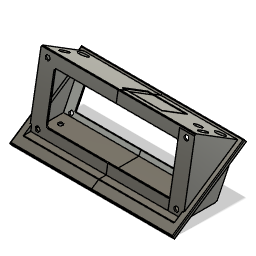
Trooper_Center_Gauges (Autodesk Fusion 360 design; units mm, degrees)
Autodesk Fusion 360 part; units mm, degrees
sketch "Base" plane through (0, 0, 0) normal (0, 1, 0) x (1, 0, 0)
  line L0 (101.6, -26.9875) -> (-101.6, -26.9875)
  line L1 (-101.6, -26.9875) -> (-101.6, 26.9875)
  line L2 (-101.6, 26.9875) -> (101.6, 26.9875)
  line L3 (101.6, 26.9875) -> (101.6, -26.9875)
  line L4 (101.6, -26.9875) -> (-101.6, 26.9875) construction
  line L5 (-101.6, -26.9875) -> (101.6, 26.9875) construction
  line L6 (-101.6, 11.7475) -> (101.6, 11.7475) construction
  circle A0 centre (-90.17, 11.7475) radius 3.175
  circle A1 centre (90.17, 11.7475) radius 3.175
  dimension "d1" = 203.2
  dimension "d2" = 53.975
  dimension "d3" = 15.24
  dimension "d4" = 6.35
  dimension "d5" = 6.35
  dimension "d6" = 11.43
  dimension "d7" = 11.43
  constraint horizontal L0
  constraint perpendicular L0 L1
  constraint parallel L0 L2
  constraint parallel L1 L3
  constraint coincident L4 origin
  constraint coincident L5 origin
  constraint coincident L1 L6.start
  constraint coincident L3 L6.end
  constraint perpendicular L3 L6
  constraint coincident L6 A0.centre
  constraint coincident L6 A1.centre
  measures "d1" distance of L1.end L2.end
  measures "d2" distance of L0.end L1.end
  measures "d3" distance of L2 L6
  measures "d4" diameter of A0
  measures "d5" diameter of A1
  measures "d6" distance of L6.start A0.centre
  measures "d7" distance of L6.end A1.centre
ref_plane "WorkPlane1" through (0, 0, -26.9875) normal (0, 0.438371, 0.898794) x (1, 0, 0)
sketch "Back" plane through (0, 0, -26.9875) normal (0, 0.438371, 0.898794) x (1, 0, 0)
  line L0 (-101.6, 0) -> (101.6, 0)
  line L1 (101.6, 0) -> (101.6, 60.325)
  line L2 (101.6, 60.325) -> (-101.6, 60.325)
  line L3 (-101.6, 60.325) -> (-101.6, 0)
  line L4 (-101.6, 0) -> (101.6, 0)
  line L5 (-88.9, 53.975) -> (88.9, 53.975)
  line L6 (88.9, 53.975) -> (88.9, 6.35)
  line L7 (88.9, 6.35) -> (-88.9, 6.35)
  line L8 (-88.9, 6.35) -> (-88.9, 53.975)
  line L9 (-101.6, 0) -> (101.6, 0)
  line L10 (101.6, 0) -> (101.6, -2.286)
  line L11 (101.6, -2.286) -> (-101.6, -2.286)
  line L12 (-101.6, -2.286) -> (-101.6, 0)
  point P0 (-101.6, 0)
  dimension "d9" = 60.325
  dimension "d10" = 12.7
  dimension "d11" = 12.7
  dimension "d12" = 6.35
  dimension "d13" = 6.35
  dimension "d28" = 2.286
  constraint horizontal L0
  constraint vertical L1
  constraint horizontal L2
  constraint vertical L3
  constraint coincident L0.end L1.start
  constraint horizontal L5
  constraint vertical L6
  constraint horizontal L7
  constraint vertical L8
  constraint coincident P0 L0.start
  constraint horizontal L9
  constraint vertical L10
  constraint horizontal L11
  constraint vertical L12
  measures "d9" distance of L2 L4
  measures "d10" distance of L3 L8
  measures "d11" distance of L1 L6
  measures "d12" distance of L2 L5
  measures "d13" distance of L0 L7
  measures "d28" distance of L9 L11
ref_plane "WorkPlane2" through (101.6, 54.2198, -53.4322) normal (0, -0.829153, -0.559022) x (1, 0, 0)
sketch "Trim" plane through (101.6, 54.2198, -53.4322) normal (0, -0.829153, -0.559022) x (1, 0, 0)
  line L0 (-203.2, 0) -> (0, 0)
  line L1 (0, 0) -> (0, 96.9903)
  line L2 (0, 96.9903) -> (-203.2, 96.9903)
  line L3 (-203.2, 96.9903) -> (-203.2, 0)
  line L4 (-211.455, -6.985) -> (8.255, -6.985)
  line L5 (8.255, -6.985) -> (8.255, 109.6903)
  line L6 (8.255, 109.6903) -> (-211.455, 109.6903)
  line L7 (-211.455, 109.6903) -> (-211.455, -6.985)
  point P0 (-203.2, 0)
  point P1 (0, 96.9903)
  point P2 (-203.2, 96.9903)
  point P3 (-203.2, 0)
  dimension "d14" = 8.255
  dimension "d15" = 8.255
  dimension "d16" = 6.985
  dimension "d17" = 12.7
  constraint horizontal L0
  constraint vertical L1
  constraint horizontal L2
  constraint vertical L3
  constraint horizontal L4
  constraint vertical L5
  constraint horizontal L6
  constraint vertical L7
  constraint coincident P2 L2.end
  constraint coincident P1 L1.end
  constraint coincident P3 P0
  measures "d14" distance of L3 L7
  measures "d15" distance of L1 L5
  measures "d16" distance of L0 L4
  measures "d17" distance of L2 L6
ref_plane "WorkPlane3" through (101.6, 0, -26.9875) normal (1, 0, 0) x (0, 1, 0)
sketch "Right" plane through (101.6, 0, -26.9875) normal (1, 0, 0) x (0, 0, -1)
  line L0 (-53.975, 0) -> (26.4447, 54.2198)
  line L1 (0, -2.032) -> (-53.975, -2.032)
  line L2 (-53.975, -2.032) -> (-53.975, 0)
  line L3 (1.8263, -0.8908) -> (28.2711, 53.329)
  line L4 (28.2711, 53.329) -> (26.4447, 54.2198)
  line L5 (0, -2.032) -> (1.8263, -0.8908)
  point P0 (26.4447, 54.2198)
  point P1 (-53.975, 0)
  dimension "d39" = 2.032
  dimension "d40" = 2.032
  constraint coincident P1 L0.start
  constraint coincident P0 L0.end
  measures "d39" distance of P1 L1.end
  measures "d40" distance of P0 L3.end
ref_plane "WorkPlane4" through (-101.6, 0, 26.9875) normal (-1, 0, 0) x (0, -1, 0)
sketch "Left" plane through (-101.6, 0, 26.9875) normal (-1, 0, 0) x (0, -1, 0)
  line L0 (0, 0) -> (-54.2198, -80.4197)
  line L1 (0.8908, -55.8013) -> (-53.329, -82.2461)
  line L2 (-53.329, -82.2461) -> (-54.2198, -80.4197)
  line L3 (2.032, -53.975) -> (2.032, 0)
  line L4 (2.032, 0) -> (0, 0)
  line L5 (0.8908, -55.8013) -> (2.032, -53.975)
  point P0 (0, -53.975)
  point P1 (-54.2198, -80.4197)
  dimension "d37" = 2.032
  dimension "d38" = 2.032
  constraint coincident L0.start L4.end
  constraint coincident P1 L0.end
  measures "d37" distance of P1 L1.end
  measures "d38" distance of L0.start L3.end
extrude "Extrude1" add sketch "Trim" along normal blind 4.572 makes body 1
extrude "Extrude2" add sketch "Back" against normal blind 2.032 contours L0 L1 L2 L3 L4 L9 bodies 1
extrude "Extrude3" add sketch "Base" against normal blind 2.032 bodies 1
extrude "Extrude4" add sketch "Right" along normal blind 2.032 bodies 1
extrude "Extrude5" add sketch "Left" along normal blind 2.032 bodies 1
extrude "Extrude6" add sketch "Back" against normal blind 2.032 contours L0 L4 L9 L10 L11 L12 bodies 1
fillet "Fillet1" radius 2.54 1 edges at (0, -2.9454, -27.8117) on bodies 1
fillet "Fillet2" radius 1.27 1 edges at (0, 0, 26.9875) on bodies 1
fillet "Fillet3" radius 1.016 4 edges at (0, -7.0996, 37.5177) (-109.855, 25.5125, -10.8531) (0, 58.1245, -59.2239) (109.855, 25.5125, -10.8531) on bodies 1
sketch "Left Tabs" plane through (-101.6, 0, 0) normal (1, 0, 0) x (0, 0, -1)
  line L0 (26.9875, 0) -> (49.4252, 46.0041)
  line L1 (49.4252, 46.0041) -> (-18.8089, 0)
  line L2 (-18.8089, 0) -> (26.9875, 0)
  line L3 (-26.67, 0) -> (-17.1035, 0) construction
  line L4 (-17.1035, 0) -> (1.1317, 103.4174) construction
  line L5 (-17.1035, 0) -> (-14.8982, 12.5071)
  line L6 (-14.8982, 12.5071) -> (-12.8971, 12.1542)
  line L7 (-12.8971, 12.1542) -> (-15.1024, -0.3529)
  line L8 (-15.1024, -0.3529) -> (-17.1035, 0)
  line L9 (-17.1035, 0) -> (-16.0009, 6.2535) construction
  line L10 (-16.0009, 6.2535) -> (-2.4932, 82.8593) construction
  line L11 (-2.4932, 82.8593) -> (-1.3905, 89.1128) construction
  line L12 (-1.3905, 89.1128) -> (-3.5959, 76.6057)
  line L13 (-3.5959, 76.6057) -> (-1.5947, 76.2529)
  line L14 (-1.5947, 76.2529) -> (0.6106, 88.7599)
  line L15 (0.6106, 88.7599) -> (-1.3905, 89.1128)
  line L16 (-26.9875, 0) -> (53.4322, 54.2198)
  line L17 (53.4322, 54.2198) -> (0.6106, 88.7599)
  line L18 (-1.5947, 76.2529) -> (-13.4282, 9.1418)
  line L19 (0.6106, 88.7599) -> (53.4322, 54.2198)
  line L20 (53.4322, 54.2198) -> (-27.3093, -0.217)
  line L21 (-27.3093, -0.217) -> (53.4322, 54.2198)
  line L22 (-36.6753, -6.5316) -> (58.3815, 57.5566)
  line L23 (58.3815, 57.5566) -> (-36.6753, -6.5316)
  line L24 (53.4322, 54.2198) -> (56.4461, 56.2518)
  line L25 (0.6106, 88.7599) -> (0.9634, 90.7611)
  line L26 (0.9634, 90.7611) -> (56.4461, 56.2518)
  line L27 (-1.3905, 89.1128) -> (-1.0377, 91.1139)
  line L28 (-1.0377, 91.1139) -> (0.9634, 90.7611)
  line L29 (-3.5959, 76.6057) -> (-14.8982, 12.5071)
  point P0 (55.2586, 53.329)
  point P1 (53.4322, 54.2198)
  point P2 (53.4322, 54.2197)
  point P3 (-36.6753, -6.5316)
  dimension "d41" = 12.7
  dimension "d42" = 2.032
  dimension "d43" = 77.7875
  dimension "d44" = 6.35
  dimension "d45" = 12.7
  dimension "d46" = 2.032
  dimension "d69" = 2.032
  dimension "d70" = 2.032
  dimension "d71" = 2.032
  dimension "d99" = 80
  dimension "d100" = 1.7054
  constraint coincident L2 L3.end
  constraint perpendicular L5 L6
  constraint parallel L5 L7
  constraint parallel L6 L8
  constraint parallel L4 L5
  constraint midpoint L5 L9.end
  constraint parallel L4 L10
  constraint parallel L4 L11
  constraint perpendicular L12 L13
  constraint parallel L12 L14
  constraint parallel L13 L15
  constraint parallel L4 L12
  constraint coincident P1 L16.end
  constraint coincident L16 L18.end
  constraint perpendicular L13 L18
  constraint coincident L22 L24.end
  constraint perpendicular L15 L25
  constraint perpendicular L15 L27
  measures "d41" distance of L3.end L5.end
  measures "d42" distance of L4 L7
  measures "d43" distance of L9.end L10.end
  measures "d44" distance of L10.end L11.end
  measures "d45" distance of L11.end L12.end
  measures "d46" distance of L10 L14
  measures "d69" vertical distance of P1 L24.end
  measures "d70" distance of L14.end L25.end
  measures "d71" distance of L11.end L27.end
  measures "d99" angle of L2 L4
  measures "d100" distance of L1.end L3.end
extrude "Extrude7" add sketch "Left Tabs" against normal blind 2.032 contours L5 L6 L7 L16 L18 L20 L21 L22 L23 | L7 L14 L16 L17 L18 L19 L20 L21 L22 L23 bodies 1
extrude "Extrude8" add sketch "Left Tabs" along normal blind 18.288 and the other way blind 2.032 contours L1 L2 L5 L7 | L1 L5 L7 L16 L20 L21 L22 L23 | L5 L6 L7 L16 L18 L20 L21 L22 L23 | L12 L13 L14 L15 bodies 1
sketch "Right Tabs" plane through (101.6, 0, 0) normal (-1, 0, 0) x (0, 0, 1)
  line L0 (-26.9875, 0) -> (26.5994, 0)
  arc A0 (27.3093, -0.217) -> (26.5994, 0) centre (26.5994, -1.27) ccw
  line L1 (27.3093, -0.217) -> (-53.4322, 54.2198)
  line L2 (-53.4322, 54.2198) -> (-26.9875, 0)
  line L3 (-53.4322, 54.2198) -> (-0.6106, 88.7599)
  line L4 (1.5947, 76.2529) -> (-0.6106, 88.7599)
  line L5 (1.5947, 76.2529) -> (13.4282, 9.1418)
  line L6 (-0.6106, 88.7599) -> (1.3905, 89.1128)
  line L7 (2.4932, 82.8593) -> (1.3905, 89.1128)
  line L8 (1.3905, 89.1128) -> (3.5959, 76.6057)
  line L9 (17.1035, 0) -> (-1.1317, 103.4174)
  line L10 (3.5959, 76.6057) -> (1.5947, 76.2529)
  line L11 (14.8982, 12.5071) -> (12.8971, 12.1542)
  line L12 (12.8971, 12.1542) -> (15.1024, -0.3529)
  line L13 (15.1024, -0.3529) -> (17.1035, 0)
  line L14 (17.1035, 0) -> (16.0009, 6.2535)
  line L15 (-1.1317, 103.4174) -> (17.1035, 0) construction
  line L16 (17.1035, 0) -> (16.0009, 6.2535) construction
  line L17 (16.0009, 6.2535) -> (2.4932, 82.8593) construction
  line L18 (2.4932, 82.8593) -> (1.3905, 89.1128) construction
  line L19 (2.4932, 82.8593) -> (3.5959, 76.6057) construction
  line L20 (-53.4322, 54.2198) -> (-0.6106, 88.7599)
  line L21 (1.3905, 89.1128) -> (3.5959, 76.6057)
  line L22 (3.5959, 76.6057) -> (1.5947, 76.2529)
  line L23 (1.5947, 76.2529) -> (-0.6106, 88.7599)
  line L24 (-0.6106, 88.7599) -> (1.3905, 89.1128)
  line L25 (14.8982, 12.5071) -> (17.1035, 0)
  line L26 (17.1035, 0) -> (15.1024, -0.3529)
  line L27 (15.1024, -0.3529) -> (12.8971, 12.1542)
  line L28 (12.8971, 12.1542) -> (14.8982, 12.5071)
  line L29 (1.5947, 76.2529) -> (13.4282, 9.1418)
  line L30 (3.5959, 76.6057) -> (14.8982, 12.5071)
  dimension "d101" = 2.032
  dimension "d102" = 2.032
  constraint coincident L9.end L15.start
  constraint coincident L9.start L13.end
  constraint coincident L14.end L16.end
  constraint coincident L7.start L17.end
  constraint coincident L6.end L7.end
  constraint coincident L8.end L10.start
  constraint coincident L1.end L2.start
  constraint coincident L3.end L4.end
  constraint perpendicular L21 L22
  constraint parallel L21 L23
  constraint parallel L22 L24
  constraint perpendicular L25 L26
  constraint parallel L25 L27
  constraint parallel L26 L28
  constraint perpendicular L13 L25
  constraint coincident L11.start L25.start
  constraint coincident L4.start L5.start
  constraint coincident L5.end L29.end
  measures "d101" distance of L18 L23
  measures "d102" distance of L15 L27
extrude "Extrude9" add sketch "Right Tabs" against normal blind 2.032 contours L1 L5 L9 L11 L12 L25 L27 L28 L29 | L1 L3 L4 L5 L12 L20 L23 L27 L29 | L5 L9 L10 L11 L22 L28 L29 L30 bodies 1
extrude "Extrude10" add sketch "Right Tabs" along normal blind 18.288 and the other way blind 2.032 contours L0 L1 L9 L12 L14 L25 L27 | L1 L5 L9 L11 L12 L25 L27 L28 L29 | L4 L6 L7 L8 L9 L10 L21 L22 L23 L24 bodies 1
extrude "Extrude12" add sketch "Left Tabs" along normal up to surface (205.232 mm away) contours L17 L19 L22 L23 L24 L25 L26 | L15 L25 L27 L28 bodies 1
ref_plane "WorkPlane5" through (-93.472, 82.5064, 0.4921) normal (0, 0.173648, 0.984808) x (0, -0.984808, 0.173648)
sketch "Tab Mounting Holes" plane through (0, 2.9249, 16.5878) normal (0, 0.173648, 0.984808) x (1, 0, 0)
  line L0 (-103.632, 74.8175) -> (-83.312, 74.8175)
  line L1 (-83.312, 74.8175) -> (-83.312, 87.5175)
  line L2 (-101.6, 87.5175) -> (-103.632, 87.5175)
  line L3 (-103.632, 87.5175) -> (-103.632, 74.8175)
  line L4 (83.312, 87.5175) -> (83.312, 74.8175)
  line L5 (83.312, 74.8175) -> (101.6, 74.8175)
  line L6 (103.632, 4.7096) -> (103.632, 87.5175)
  line L7 (-101.6, 4.7097) -> (-101.6, -1.6449)
  line L8 (-101.6, -1.6449) -> (-101.6, -2.97)
  line L9 (-101.6, -2.97) -> (-83.312, -2.97)
  line L10 (-83.312, -2.97) -> (-83.312, 9.73)
  line L11 (-83.312, 9.73) -> (-103.632, 9.73)
  line L12 (101.6, 74.8175) -> (101.6, 9.73)
  line L13 (83.312, 87.5175) -> (83.312, 74.8175)
  line L14 (83.312, -2.97) -> (101.6, -2.97)
  line L15 (-103.632, 9.73) -> (-83.312, -2.97) construction
  circle A0 centre (-93.472, 81.1675) radius 3.175
  circle A1 centre (-93.472, 3.38) radius 3.175
  line L16 (-83.312, 87.5175) -> (83.312, 87.5175)
  line L17 (83.312, 87.5175) -> (103.632, 87.5175)
  line L18 (103.632, 87.5175) -> (103.632, 89.5495)
  line L19 (103.632, 89.5495) -> (-101.6, 89.5495)
  line L20 (-101.6, 89.5495) -> (-101.6, 87.5175)
  line L21 (103.632, 87.5175) -> (83.312, 87.5175)
  line L22 (101.6, 74.8175) -> (101.6, 9.73)
  line L23 (101.6, 4.7096) -> (103.632, 4.7096)
  line L24 (101.6, 74.8175) -> (103.632, 74.8175) construction
  line L25 (-103.632, 9.73) -> (-103.632, 4.7097)
  line L26 (-103.632, 4.7096) -> (-101.6, 4.7096)
  line L27 (101.6, 9.73) -> (83.312, 9.73)
  line L28 (83.312, 9.73) -> (83.312, -2.97)
  line L29 (83.312, -2.97) -> (101.6, -2.97)
  line L30 (101.6, -2.97) -> (101.6, 4.7096)
  line L31 (103.632, 4.7096) -> (103.632, 87.5175)
  line L32 (103.632, 87.5175) -> (83.312, 87.5175)
  line L33 (83.312, 74.8175) -> (101.6, 74.8175)
  line L34 (101.6, 9.73) -> (83.312, 9.73)
  line L35 (83.312, 9.73) -> (83.312, -2.97)
  line L36 (101.6, -2.97) -> (101.6, 4.7096)
  line L37 (101.6, 4.7096) -> (103.632, 4.7096)
  line L38 (-83.312, 74.8175) -> (-103.632, 87.5175) construction
  line L39 (-83.312, 87.5175) -> (-103.632, 74.8175) construction
  line L40 (103.632, 87.5175) -> (83.312, 74.8175) construction
  line L41 (83.312, 87.5175) -> (103.632, 74.8175) construction
  line L42 (-101.6, -2.97) -> (-103.632, -2.97) construction
  line L43 (-103.632, -2.97) -> (-103.632, 4.7096) construction
  line L44 (101.6, -2.97) -> (103.632, -2.97) construction
  line L45 (103.632, 4.7096) -> (103.632, -2.97) construction
  line L46 (83.312, 9.73) -> (103.632, -2.97) construction
  line L47 (101.6, 9.73) -> (103.632, 9.73) construction
  line L48 (83.312, -2.97) -> (103.632, 9.73) construction
  line L49 (-83.312, 9.73) -> (-103.632, -2.97) construction
  circle A2 centre (93.472, 81.1675) radius 3.175
  circle A3 centre (93.472, 3.38) radius 3.175
  point P0 (-93.472, 3.38)
  point P1 (-93.472, 81.1675)
  point P2 (93.472, 81.1675)
  point P3 (93.472, 3.38)
  dimension "d60" = 77.7875
  dimension "d62" = 6.35
  dimension "d63" = 6.35
  dimension "d104" = 2.032
  dimension "d105" = 2.032
  dimension "d106" = 2.032
  dimension "d107" = 6.35
  dimension "d108" = 6.35
  constraint coincident L11.end L15.start
  constraint coincident L9.end L10.start
  constraint midpoint L15 P0
  constraint coincident P1 A0.centre
  constraint coincident P0 A1.centre
  constraint coincident L5.end L12.start
  constraint coincident L6 L24.end
  constraint perpendicular L6 L24
  constraint coincident L0.end L1.start
  constraint coincident L2.end L3.start
  constraint coincident L1.end L16.start
  constraint coincident L0.start L3.end
  constraint coincident L6.end L17.end
  constraint coincident L4.end L5.start
  constraint coincident L4.start L13.start
  constraint midpoint L41 P2
  constraint coincident L8.end L9.start
  constraint perpendicular L8 L42
  constraint coincident L26.start L43.end
  constraint coincident L14.end L29.end
  constraint perpendicular L30 L44
  constraint coincident L6.start L23.end
  constraint coincident L27.end L28.start
  constraint coincident L12.end L22.end
  constraint perpendicular L6 L47
  constraint coincident L14.start L28.end
  constraint coincident L10.end L11.start
  constraint midpoint L46 P3
  constraint coincident P2 A2.centre
  constraint coincident P3 A3.centre
  measures "d60" vertical distance of P0 P1
  measures "d62" diameter of A0
  measures "d63" diameter of A1
  measures "d104" distance of L8.end L42.end
  measures "d105" distance of L14.end L44.end
  measures "d106" distance of L12.end L47.end
  measures "d107" diameter of A2
  measures "d108" diameter of A3
extrude "Extrude11" cut sketch "Tab Mounting Holes" against normal blind 2.032 contours A0 | A1 | A2 | A3 bodies 1
extrude "Extrude20" cut sketch "Tab Mounting Holes" against normal through all contours A0 | A2 bodies 1
extrude "Extrude13" add sketch "Left Tabs" against normal up to surface (2.032 mm away) contours L17 L19 L22 L23 L24 L25 L26 | L15 L25 L27 L28 bodies 1
sketch "Screwdriver Holes - Back" plane through (0, -11.524, -23.6277) normal (0, -0.438371, -0.898794) x (-1, 0, 0)
  line L0 (-103.632, 12.0332) -> (101.6, 12.0332)
  line L1 (101.6, 12.0332) -> (101.6, 66.5327)
  line L2 (101.6, 66.5327) -> (101.6, 70.9818)
  line L3 (101.6, 70.9818) -> (-101.6, 70.9818)
  line L4 (-101.6, 70.9818) -> (-101.6, 66.5327)
  line L5 (-101.6, 66.5327) -> (-103.632, 66.5327)
  line L6 (-103.632, 66.5327) -> (-103.632, 12.0332)
  line L7 (88.9, 18.1805) -> (-88.9, 18.1805)
  line L8 (-88.9, 18.1805) -> (-88.9, 65.8055)
  line L9 (-88.9, 65.8055) -> (88.9, 65.8055)
  line L10 (88.9, 65.8055) -> (88.9, 18.1805)
  line L11 (-92.964, 15.24) -> (92.7862, 15.24) construction
  circle A0 centre (-92.964, 15.24) radius 2.794
  circle A1 centre (92.7862, 15.24) radius 2.794
  dimension "d111" = 185.7502
  dimension "d113" = 4.064
  dimension "d114" = 5.588
  dimension "d115" = 5.588
  constraint perpendicular L8 L11
  constraint coincident L11.start A0.centre
  constraint coincident L11.end A1.centre
  measures "d111" distance of L11.start L11.end
  measures "d113" horizontal distance of L7.end L11.start
  measures "d114" diameter of A0
  measures "d115" diameter of A1
extrude "Extrude21" cut sketch "Screwdriver Holes - Back" against normal blind 2.032 contours A0 | A1 bodies 1
ref_plane "WorkPlane6" through (0, 0, -11.7475) normal (0, -0.45399, -0.891007) x (1, 0, 0)
ref_plane "WorkPlane7" through (0, 73.5064, -28.7048) normal (0, 0.849148, -0.528156) x (0, 0.528156, 0.849148)
sketch "Screwdriver Holes - Top" plane through (0, 73.5064, -28.7048) normal (0, 0.849148, -0.528156) x (0, 0.528156, 0.849148)
  line L0 (32.6696, 103.632) -> (-32.6696, 103.632)
  line L1 (-32.6696, -103.632) -> (32.6696, -103.632)
  line L2 (-18.3286, 180.8064) -> (-18.3286, -180.8064)
  line L3 (-18.3286, 103.632) -> (-18.3286, 92.202) construction
  line L4 (-18.3286, -103.632) -> (-18.3286, -92.202) construction
  circle A0 centre (-18.3286, -92.202) radius 6.35
  circle A1 centre (-18.3286, 92.202) radius 6.35
  point P0 (-24.4236, 90.17)
  point P1 (-24.4236, -90.17)
  dimension "d78" = 11.43
  dimension "d79" = 11.43
  dimension "d80" = 12.7
  dimension "d81" = 12.7
  constraint coincident L2 L3.start
  constraint coincident L0 L3.start
  constraint coincident L2 L3.end
  constraint coincident L1 L4.start
  constraint coincident L2 L4.start
  constraint coincident L2 L4.end
  constraint coincident L4.end A0.centre
  constraint coincident L3.end A1.centre
  measures "d78" distance of L3.start L3.end
  measures "d79" distance of L4.start L4.end
  measures "d80" diameter of A0
  measures "d81" diameter of A1
extrude "Extrude14" cut sketch "Screwdriver Holes - Top" along normal up to surface end surface through (-101.6, 54.2198, -53.4322) normal (0, -0.836948, 0.547282) offset 0 bodies 1
sketch "Tab Connector Left" plane through (0, 73.6809, -12.9919) normal (0, -0.984808, 0.173648) x (1, 0, 0)
  line L0 (-101.6, 14.8117) -> (-83.312, 14.8117)
  line L1 (-83.312, 14.8117) -> (-83.312, 16.8437)
  line L2 (-83.312, 16.8437) -> (-103.632, 16.8437)
  line L3 (-103.632, 14.8117) -> (-101.6, 14.8117)
  line L4 (-103.632, 16.8437) -> (-103.632, 14.8117)
sketch "Tab Connector Bottom" plane through (-83.312, 0, 0) normal (1, 0, 0) x (0, 0, -1)
  line L0 (-17.1035, 0) -> (-15.0402, 0)
  line L1 (-15.0402, 0) -> (-12.8971, 12.1542)
  line L2 (-12.8971, 12.1542) -> (-14.8982, 12.5071)
  line L3 (-14.8982, 12.5071) -> (-17.1035, 0)
sketch "Tab Connector Top" plane through (-83.312, 0, 0) normal (1, 0, 0) x (0, 0, -1)
  line L0 (0.6106, 88.7599) -> (-1.3905, 89.1128)
  line L1 (-1.3905, 89.1128) -> (-3.5959, 76.6057)
  line L2 (-3.5959, 76.6057) -> (-1.5947, 76.2529)
  line L3 (-1.5947, 76.2529) -> (0.6106, 88.7599)
sketch "Tab Connector Right" plane through (0, 73.6809, -12.9919) normal (0, -0.984808, 0.173648) x (1, 0, 0)
  line L0 (101.6, 14.8117) -> (101.6, 16.8437)
  line L1 (101.6, 16.8437) -> (83.312, 16.8437)
  line L2 (83.312, 14.8117) -> (101.6, 14.8117)
  line L3 (83.312, 16.8437) -> (83.312, 14.8117)
extrude "Extrude16" add sketch "Tab Connector Bottom" along normal up to surface (166.624 mm away) bodies 1
extrude "Extrude19" add sketch "Tab Connector Left" along normal up to surface (65.0875 mm away) bodies 1
extrude "Extrude17" add sketch "Tab Connector Top" along normal up to surface (166.624 mm away) bodies 1
extrude "Extrude18" add sketch "Tab Connector Right" along normal up to surface (65.0875 mm away) bodies 1
fillet "Fillet5" radius 2.54 4 edges at (-83.312, 76.4293, 2.5953) (83.312, 76.4293, 2.5953) (83.312, 12.3306, 13.8976) (-83.312, 12.3306, 13.8976) on bodies 1
sketch "GPS Mount" plane through (0, 65.8755, -40.9735) normal (0, 0.849148, -0.528156) x (-1, 0, 0)
  circle A0 centre (-92.202, -3.8804) radius 6.35
  circle A1 centre (92.202, -3.8804) radius 6.35
  ellipse E0 centre (93.472, 24.6267) end of major axis (93.472, 16.1073) minor radius 3.175
  ellipse E1 centre (-93.472, 24.6266) end of major axis (-93.472, 16.1072) minor radius 3.175
  line L0 (-103.632, 47.1179) -> (-103.632, -18.2214)
  line L1 (-103.632, -18.2214) -> (103.632, -18.2214)
  line L2 (103.632, -18.2214) -> (103.632, 47.1179)
  line L3 (103.632, 47.1179) -> (-103.632, 47.1179)
  line L4 (-78.232, -18.2214) -> (-78.232, 47.1179) construction
  circle A2 centre (-78.232, 14.2906) radius 5.08
  line L5 (-78.232, 14.2906) -> (-59.182, 14.2906) construction
  line L6 (-59.182, 14.2906) -> (-19.812, 14.2906) construction
  line L7 (6.858, 34.6106) -> (-46.482, 34.6106)
  line L8 (-46.482, 34.6106) -> (-46.482, -6.0294)
  line L9 (-46.482, -6.0294) -> (6.858, -6.0294)
  line L10 (6.858, -6.0294) -> (6.858, 34.6106)
  line L11 (6.858, 34.6106) -> (-46.482, -6.0294) construction
  line L12 (-46.482, 34.6106) -> (6.858, -6.0294) construction
  point P0 (-78.232, 14.2906)
  point P1 (-19.812, 14.2906)
  dimension "d118" = 25.4
  dimension "d120" = 32.512
  dimension "d121" = 10.16
  dimension "d122" = 19.05
  dimension "d123" = 39.37
  dimension "d124" = 53.34
  dimension "d125" = 40.64
  constraint coincident L1 L4.start
  constraint coincident L3 L4.end
  constraint perpendicular L3 L4
  constraint coincident L4 P0
  constraint coincident P0 A2.centre
  constraint perpendicular L4 L5
  constraint parallel L5 L6
  constraint horizontal L7
  constraint perpendicular L7 L8
  constraint parallel L7 L9
  constraint parallel L8 L10
  constraint coincident L11 P1
  constraint coincident L12 P1
  constraint coincident P1 L6.end
  measures "d118" distance of L0 L4
  measures "d120" distance of L1 P0
  measures "d121" diameter of A2
  measures "d122" distance of P0 L5.end
  measures "d123" distance of L5.end P1
  measures "d124" distance of L8.end L9.end
  measures "d125" distance of L7.end L8.end
extrude "Extrude22" cut sketch "GPS Mount" against normal blind 0.762 contours L7 L8 L9 L10 bodies 1
extrude "Extrude23" cut sketch "GPS Mount" against normal blind 3.81 contours A2 bodies 1
ref_plane "WorkPlane10" through (0, 23.1958, -12.415) normal (-1, 0, 0) x (0, 0.559022, -0.829153)
split "Split4" by plane through (0, 23.1958, -12.415) normal (-1, 0, 0) bodies 1 makes body 2 at (-33.3356, 70.6325, -33.3253)
equation "d43 = 3 1/16\""
named bodies: "Trooper_Gauge_Insert_R", "Trooper_Gauge_Insert_L"
